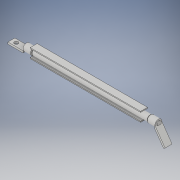
# Autodesk Inventor part: Cable Primitive
Saved by Autodesk Inventor 2017 (Build 210142000, 142)
## iProperties
Created: 2021-03-10
Part Number: Cable Primitive
Material: Generic
Document SubType Name: Modeling
Designer: Win240
Density: 1 g/cm^3
Appearance: Default
Author: Win240
Autodesk Inventor part; units mm, degrees
ref_plane "YZ Plane" through (0, 0, 0) normal (1, 0, 0) x (0, 1, 0)
sketch "Sketch1" plane through (0, 0, 0) normal (0, 0, 1) x (1, 0, 0)
  line L0 (-76.2, -2) -> (76.2, -2)
  line L1 (76.2, 2) -> (-76.2, 2)
  line L2 (-76.2, -2) -> (76.2, 2) construction
  line L3 (76.2, -2) -> (-76.2, 2) construction
  line L4 (-76.2, -2) -> (-76.2, -0.85)
  line L5 (-76.2, -0.85) -> (-88.2, -0.85)
  line L6 (-88.2, -0.85) -> (-88.2, 2)
  line L7 (-88.2, 2) -> (-76.2, 2)
  line L8 (76.2, -2) -> (76.2, -0.85)
  line L9 (76.2, -0.85) -> (88.2, -0.85)
  line L10 (88.2, -0.85) -> (88.2, 2)
  line L11 (88.2, 2) -> (76.2, 2)
  point P0 (0, 0)
  point P1 (0, 0)
  point P2 (0, 0)
  dimension "d3" = 4
  dimension "d4" = 2.85
  dimension "d5" = 12
  dimension "d6" = 152.4
  constraints: 24 end point, 5 horizontal, 4 vertical, 3 midpoint, 2 coincident, 2 equal length, 1 collinear, 1 parallel
  measures "d3" distance between parallel lines of L1 L0
  measures "d4" distance of L5.end L6.end
  measures "d5" distance of L4.end L5.end
  measures "d6" distance of L0.start L0.end
revolve "Revolution1" add sketch "Sketch1" angle 360 about axis through (76.2, 2, 0) along (-1, 0, 0)
ref_plane "Work Plane1" through (-77.7, 2, 0) normal (-1, 0, 0) x (0, 0, 1)
sketch "Sketch2" plane through (-77.7, 2, 0) normal (-1, 0, 0) x (0, 0, 1)
  circle A0 centre (0, 0) radius 2.85 projected
  circle A1 centre (0, 0) radius 4.6
  point P0 (0, -2)
  dimension "d9" = 9.2
  constraints: 1 centre point, 1 coincident
  measures "d9" diameter of A1
extrude "Extrusion1" add sketch "Sketch2" along normal blind 10
ref_plane "Work Plane2" through (77.2, 2, 0) normal (1, 0, 0) x (0, 0, -1)
sketch "Sketch3" plane through (77.2, 2, 0) normal (1, 0, 0) x (0, 0, -1)
  circle A0 centre (0, 0) radius 4.6 projected
  point P0 (0, -2)
extrude "Extrusion2" add sketch "Sketch3" along normal blind 10
sketch "Sketch4" plane through (0, 0, 0) normal (0, 1, 0) x (-1, 0, 0)
  line L0 (87.7, -4.6) -> (87.7, 4.6) projected
  line L1 (-87.2, 4.6) -> (-87.2, -4.6) projected
  line L2 (87.7, 4.6) -> (107.7, 4.6)
  line L3 (107.7, 4.6) -> (107.7, -4.6)
  line L4 (107.7, -4.6) -> (87.7, -4.6)
  point P0 (0, 0)
  dimension "d15" = 20
  constraints: 6 end point, 2 horizontal, 1 vertical
  measures "d15" distance of L0.end L2.end
extrude "Extrusion3" add sketch "Sketch4" against normal blind 2.5
sketch "Sketch5" plane through (-107.7, 0, 4.6) normal (0, 0, 1) x (1, 0, 0)
  line L0 (194.9, -2.6) -> (194.9, 6.6) projected
  line L1 (194.9, -2.6) -> (206.3715, -18.983)
  line L2 (206.3715, -18.983) -> (208.4194, -17.5491)
  line L3 (208.4194, -17.5491) -> (194.9, 1.7586)
  line L4 (0, 0) -> (0, -2.5) construction
  line L5 (20, -2.5) -> (0, -2.5) construction
  point P0 (107.7, 0)
  dimension "d18" = 145
  constraints: 6 end point, 2 equal length, 2 perpendicular, 1 point on line
  measures "d18" angle of L0 L1
extrude "Extrusion4" add sketch "Sketch5" against normal up to surface (9.2 mm away)
sketch "Sketch6" plane through (-107.7, 0, 4.6) normal (0, 0, 1) x (1, 0, 0)
  line L0 (30, 6.6) -> (20, 6.6) construction
  line L1 (30, -2.6) -> (20, -2.6) construction
  line L2 (19.5, 4.85) -> (19.5, 0) construction
  line L3 (195.9, 4.85) -> (195.9, 0.3305) construction
  line L4 (29.5, 8.35) -> (175.9, 8.35)
  line L5 (175.9, 8.35) -> (175.9, 7.08)
  line L6 (175.9, 7.08) -> (29.5, 7.08)
  line L7 (29.5, 7.08) -> (29.5, 8.35)
  line L8 (29.5, -3.08) -> (175.9, -3.08)
  line L9 (175.9, -3.08) -> (175.9, -4.35)
  line L10 (175.9, -4.35) -> (29.5, -4.35)
  line L11 (29.5, -4.35) -> (29.5, -3.08)
  line L12 (25, -2.6) -> (25, -3.08) construction
  line L13 (25, 6.6) -> (25, 7.08) construction
  point P0 (107.7, 0)
  dimension "d21" = 12.7
  dimension "d22" = 1.27
  dimension "d23" = 20
  dimension "d26" = 10
  constraints: 20 end point, 4 parallel, 3 collinear, 3 point on line, 2 horizontal, 2 midpoint, 2 perpendicular, 2 vertical
  measures "d21" distance between parallel lines of L10 L4
  measures "d22" distance of L6.end L4.start
  measures "d23" distance between parallel lines of L3 L5
  measures "d26" distance between parallel lines of L7 L2
extrude "Extrusion5" add sketch "Sketch6" against normal up to surface (9.2 mm away)
sketch "Sketch7" plane through (0, 0, 0) normal (0, 1, 0) x (1, 0, 0)
  line L0 (-88.2, 2.0304) -> (-88.2, -2.0304) construction
  line L1 (-88.2, 0) -> (-101.2, 0) construction
  circle A0 centre (-101.2, 0) radius 2.5
  point P0 (0, 0)
  dimension "d27" = 5
  dimension "d28" = 13
  constraints: 2 end point, 1 centre point, 1 coincident, 1 horizontal, 1 midpoint
  measures "d27" diameter of A0
  measures "d28" distance of L1.start L1.end
extrude "Extrusion6" cut sketch "Sketch7" against normal up to surface (2.5 mm away)
body "Solid1"
